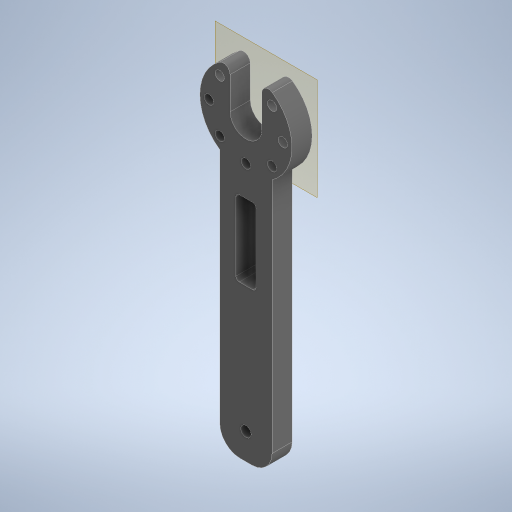
# Autodesk Inventor part: 7
Saved by Autodesk Inventor 2024.3 (Build 283343000, 343)
## iProperties
Created: 2024-09-05
Part Number: 7
Material: 아크릴, 선명
Document SubType Name: Modeling
Designer: 구지현
Density: 1.19 g/cm^3
Appearance: 회색
Mass: 8.95754 g
Surface Area: 51.4889 cm^2
Volume: 7.52734 cm^3
Author: 구지현
Autodesk Inventor part; units mm, degrees
ref_plane "YZ Plane" through (0, 0, 0) normal (1, 0, 0) x (0, 1, 0)
ref_plane "XZ Plane" through (0, 0, 0) normal (0, 1, 0) x (-1, 0, 0)
ref_plane "XY Plane" through (0, 0, 0) normal (0, 0, 1) x (1, 0, 0)
ref_plane "작업 평면1" through (0, 0, 0) normal (0, 0, 1) x (1, 0, 0)
sketch "스케치1" plane through (0, 0, 0) normal (0, 0, 1) x (1, 0, 0)
  circle A0 centre (0, 0) radius 13.8 projected
  circle A1 centre (0, 0) radius 7.2 projected
  circle A2 centre (0, -11) radius 1.2812 projected
  circle A3 centre (-7.7782, -7.7782) radius 1.2812 projected
  circle A4 centre (-11, 0) radius 1.2812 projected
  circle A5 centre (-7.7782, 7.7782) radius 1.2812 projected
  circle A6 centre (0, 11) radius 1.2812 projected
  circle A7 centre (7.7782, 7.7782) radius 1.2812 projected
  circle A8 centre (11, 0) radius 1.2812 projected
  circle A9 centre (7.7782, -7.7782) radius 1.2812 projected
  circle A10 centre (0, 0) radius 6 projected
  circle A11 centre (0, 0) radius 4.6 projected
  circle A12 centre (7.7782, -7.7782) radius 1.3812
  circle A13 centre (11, 0) radius 1.3812
  circle A14 centre (7.7782, 7.7782) radius 1.3812
  circle A15 centre (0, 11) radius 1.3812
  circle A16 centre (-7.7782, 7.7782) radius 1.3812
  circle A17 centre (-11, 0) radius 1.3812
  circle A18 centre (-7.7782, -7.7782) radius 1.3812
  circle A19 centre (0, -11) radius 1.3812
  arc A20 (-4.7, 0) -> (4.7, 0) centre (0, 0) ccw
  line L0 (4.7, 0) -> (4.7, 9.5917)
  line L1 (-4.7, 0) -> (-4.7, 9.5917)
  arc A21 (-4.7, 9.5917) -> (-7.8453, 11.2313) centre (-6.7, 9.5917) ccw
  arc A22 (7.8453, 11.2313) -> (4.7, 9.5917) centre (6.7, 9.5917) ccw
  line L2 (-7.7782, -11.2779) -> (-7.7782, -56.7782)
  line L3 (-1.7782, -62.7782) -> (1.7782, -62.7782)
  arc A23 (1.7782, -62.7782) -> (7.7782, -56.7782) centre (1.7782, -56.7782) ccw
  arc A24 (-7.7782, -56.7782) -> (-1.7782, -62.7782) centre (-1.7782, -56.7782) ccw
  arc A25 (-7.8453, 11.2313) -> (-7.7782, -11.2779) centre (0, 0) ccw
  arc A26 (7.7782, -11.2779) -> (7.8453, 11.2313) centre (0, 0) ccw
  line L4 (7.7782, -11.2779) -> (7.7782, -56.7782)
  line L5 (0, -62.7782) -> (0, -56.7782)
  circle A27 centre (0, -56.7782) radius 1.55
  line L6 (0, 0) -> (0, -55)
  line L7 (0, 0) -> (55, 0) construction
  circle A28 centre (0, -55) radius 1.55
  point P0 (4.7, 12.8686)
  point P1 (-4.7, 12.8686)
  point P2 (7.7782, -62.7782)
  point P3 (-7.7782, -62.7782)
  dimension "d1" = 0.1
  dimension "d2" = 0.1
  dimension "d3" = 0.1
  dimension "d4" = 0.1
  dimension "d5" = 0.1
  dimension "d6" = 0.1
  dimension "d7" = 0.1
  dimension "d8" = 0.1
  dimension "d9" = 0.1
  dimension "d10" = 2
  dimension "d11" = 55
  dimension "d12" = 55
  dimension "d13" = 6
  dimension "d16" = 6
  dimension "d17" = 3.1
  dimension "d18" = 55
  dimension "d19" = 90
  dimension "d20" = 3.1
  constraints: 17 centre point, 16 end point, 14 point on circle, 8 tangent, 5 point on line, 5 vertical, 2 coincident, 2 equal radius, 1 collinear, 1 horizontal, 1 midpoint, 1 perpendicular
  measures "d1" radial gap between concentric circles of A9 A12
  measures "d2" radial gap between concentric circles of A8 A13
  measures "d3" radial gap between concentric circles of A7 A14
  measures "d4" radial gap between concentric circles of A6 A15
  measures "d5" radial gap between concentric circles of A5 A16
  measures "d6" radial gap between concentric circles of A4 A17
  measures "d7" radial gap between concentric circles of A3 A18
  measures "d8" radial gap between concentric circles of A2 A19
  measures "d9" radial gap between concentric circles of A11 A20
  measures "d10" radius of A21
  measures "d11" distance of A9.centre point (7.778, -62.778)
  measures "d12" distance of A3.centre point (-7.778, -62.778)
  measures "d13" radius of A23
  measures "d16" distance of L5.start L5.end
  measures "d17" diameter of A27
  measures "d18" distance of L6.start L6.end
  measures "d19" angle of L6 L7
  measures "d20" diameter of A28
extrude "돌출1" add sketch "스케치1" along normal blind 6 contours L2 A25 A21 L1 A1 L6 A19 A0 | A0 L6 A28 A27 L5 L3 A24 L2 | L4 A23 L3 L5 A27 A28 L6 A0 | A0 L6 A19 A1 L0 A22 A26 L4 | A28 A27 | L6 A10 L0 A1 | A1 L1 A10 L6 | L6 A20 L0 A10 | A10 L1 A20 L6 picked at (-0.124, -57.7204)
move faces "이동1" translate (0, -25, 0) faces at (1.5299, -55.2486, 4) (-6.7356, -60.1581, 4) (6.7356, -60.1581, 4) (-0.5927, -62.7782, 2)
sketch "스케치2" plane through (0, 0, 6) normal (0, 0, 1) x (1, 0, 0)
  arc A0 (-7.7782, -81.7782) -> (-1.7782, -87.7782) centre (-1.7782, -81.7782) ccw projected
  line L0 (-1.7782, -87.7782) -> (1.7782, -87.7782) projected
  arc A1 (1.7782, -87.7782) -> (7.7782, -81.7782) centre (1.7782, -81.7782) ccw projected
  line L1 (7.7782, -81.7782) -> (7.7782, -11.2779) projected
  arc A2 (7.7782, -11.2779) -> (7.8453, 11.2313) centre (0, 0) ccw projected
  arc A3 (7.8453, 11.2313) -> (4.7, 9.5917) centre (6.7, 9.5917) ccw projected
  line L2 (4.7, 9.5917) -> (4.7, 0) projected
  arc A4 (-4.7, 0) -> (4.7, 0) centre (0, 0) ccw projected
  line L3 (-4.7, 0) -> (-4.7, 9.5917) projected
  arc A5 (-4.7, 9.5917) -> (-7.8453, 11.2313) centre (-6.7, 9.5917) ccw projected
  arc A6 (-7.8453, 11.2313) -> (-7.7782, -11.2779) centre (0, 0) ccw projected
  line L4 (-7.7782, -11.2779) -> (-7.7782, -81.7782) projected
  circle A7 centre (0, -11) radius 1.3812 projected
  circle A8 centre (7.7782, -7.7782) radius 1.3812 projected
  circle A9 centre (11, 0) radius 1.3812 projected
  circle A10 centre (7.7782, 7.7782) radius 1.3812 projected
  circle A11 centre (-7.7782, 7.7782) radius 1.3812 projected
  circle A12 centre (-11, 0) radius 1.3812 projected
  circle A13 centre (-7.7782, -7.7782) radius 1.3812 projected
  circle A14 centre (0, -80) radius 1.55 projected
  line L5 (0, -11) -> (0, -20)
  line L6 (0, -11) -> (9, -11) construction
  circle A15 centre (0, -80) radius 1.55 projected
  line L7 (0, -80) -> (0, -71)
  line L8 (0, -71) -> (-3, -71)
  line L9 (0, -71) -> (3, -71)
  line L10 (-3, -71) -> (3, -71)
  line L11 (3, -71) -> (3, -20)
  line L12 (3, -20) -> (-3, -20)
  line L13 (-3, -20) -> (-3, -71)
  line L14 (0, -71) -> (0, -20)
  line L15 (0, -71) -> (0, -45.5)
  line L16 (0, -45.5) -> (0, -20)
  line L17 (0, -45.5) -> (0, -42.5)
  line L18 (0, -45.5) -> (0, -48.5)
  line L19 (-3, -48.5) -> (3, -48.5)
  line L20 (3, -48.5) -> (3, -42.5)
  line L21 (3, -42.5) -> (-3, -42.5)
  line L22 (-3, -42.5) -> (-3, -48.5)
  dimension "d30" = 9
  dimension "d31" = 90
  dimension "d32" = 9
  dimension "d33" = 3
  dimension "d34" = 3
  dimension "d38" = 51
  dimension "d39" = 25.5
  dimension "d40" = 3
  dimension "d41" = 3
  constraints: 36 end point, 5 parallel, 5 perpendicular, 4 horizontal, 4 point on line, 2 vertical, 1 midpoint
  measures "d30" distance of L5.start L5.end
  measures "d31" angle of L5 L6
  measures "d32" distance of L7.start L7.end
  measures "d33" distance of L7.end L8.end
  measures "d34" distance of L7.end L9.end
  measures "d38" distance of L7.end L5.end
  measures "d39" distance of L7.end L15.end
  measures "d40" distance of L15.end L17.end
  measures "d41" distance of L15.end L18.end
extrude "돌출2" cut sketch "스케치2" against normal blind 10 contours L13 L12 L14 L21 | L21 L14 L12 L11
fillet "모깎기1" radius 1 2 edges at (-3, -20, 3) (3, -20, 3)
fillet "모깎기2" radius 1 2 edges at (3, -42.5, 3) (-3, -42.5, 3)
